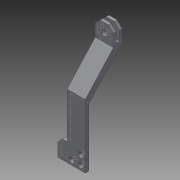
# Autodesk Inventor part: col support base
Saved by Autodesk Inventor 2015 (Build 190159000, 159)
## iProperties
Created: 2019-01-13
Part Number: col support base
Material: Generic
Document SubType Name: Modeling
Designer: Toby
Density: 1 g/cm^3
Appearance: Default
Author: Toby
Autodesk Inventor part; units mm, degrees
ref_plane "YZ Plane" through (0, 0, 0) normal (1, 0, 0) x (0, 1, 0)
ref_plane "XZ Plane" through (0, 0, 0) normal (0, 1, 0) x (-1, 0, 0)
ref_plane "XY Plane" through (0, 0, 0) normal (0, 0, 1) x (1, 0, 0)
sketch "Sketch1" plane through (0, 0, 0) normal (0, 0, 1) x (1, 0, 0)
  line L0 (-18.6815, -3.2252) -> (11.3185, -3.2252)
  line L1 (11.3185, -3.2252) -> (11.3185, -7.2252)
  line L2 (11.3185, -7.2252) -> (-18.6815, -7.2252)
  line L3 (-18.6815, -7.2252) -> (-18.6815, -3.2252)
  point P0 (0, 0)
  dimension "d0" = 30
  dimension "d1" = 4
  constraints: 8 end point, 2 parallel, 1 horizontal, 1 perpendicular
  measures "d0" distance of L0.start L0.end
  measures "d1" distance of L2.end L0.start
extrude "Extrusion1" add sketch "Sketch1" along normal blind 20
sketch "Sketch2" plane through (-18.6815, -7.2252, 0) normal (0, -1, 0) x (1, 0, 0)
  line L0 (30, 20) -> (10, 20)
  line L1 (10, 20) -> (10, 123)
  line L2 (10, 123) -> (30, 123)
  line L3 (30, 123) -> (30, 20)
  point P0 (18.6815, 0)
  dimension "d4" = 103
  dimension "d5" = 20
  constraints: 8 end point, 2 parallel, 1 horizontal, 1 perpendicular
  measures "d4" distance of L0.end L1.end
  measures "d5" distance of L1.end L2.end
extrude "Extrusion2" add sketch "Sketch2" against normal blind 10
sketch "Sketch3" plane through (-18.6815, -7.2252, 0) normal (0, -1, 0) x (1, 0, 0)
  line L0 (30, 20) -> (10, 20) projected
  line L1 (30, 0) -> (30, 20) projected
  line L2 (30, 0) -> (0, 0) projected
  point P0 (18.6815, 0)
  point P1 (25, 15)
  point P2 (25, 5)
  point P3 (15, 5)
  dimension "d8" = 5
  dimension "d9" = 5
  dimension "d10" = 5
  dimension "d11" = 5
  dimension "d12" = 5
  dimension "d13" = 10
  measures "d8" distance from line of L0 point (25, 15)
  measures "d9" distance from line of L1 point (25, 15)
  measures "d10" distance from line of L2 point (25, 5)
  measures "d11" distance from line of L1 point (25, 5)
  measures "d12" distance from line of L2 point (15, 5)
  measures "d13" distance of point (25, 5) point (15, 5)
hole "Hole1" at (6.3185, -7.2252, 15) at (6.3185, -7.2252, 5) at (-3.6815, -7.2252, 5) direction (0, 1, 0) diameter 3 depth 8 tip angle 118 countersink diameter 6 countersink angle 90
chamfer "Chamfer1" distance 5 angle 45 1 edges at (-18.6815, -5.2252, 20)
sketch "Sketch4" plane through (-8.6815, -7.2252, 20) normal (-1, 0, 0) x (0, 0, 1)
  line L0 (103, 10) -> (0, 10)
  line L1 (0, 10) -> (0, 4)
  line L2 (0, 4) -> (103, 4)
  line L3 (103, 4) -> (103, 10)
  point P0 (-20, 7.2252)
  constraints: 8 end point, 2 parallel, 1 horizontal, 1 perpendicular
extrude "Extrusion3" cut sketch "Sketch4" against normal blind 20
sketch "Sketch5" plane through (-8.6815, -7.2252, 20) normal (-1, 0, 0) x (0, 0, 1)
  line L0 (103, 4) -> (99, 4)
  line L1 (99, 4) -> (99, 34)
  line L2 (99, 34) -> (103, 34)
  line L3 (103, 34) -> (103, 4)
  point P0 (-20, 7.2252)
  dimension "d26" = 4
  dimension "d27" = 30
  constraints: 8 end point, 2 parallel, 1 horizontal, 1 perpendicular
  measures "d26" distance between parallel lines of L1 L3
  measures "d27" distance between parallel lines of L0 L2
extrude "Extrusion4" add sketch "Sketch5" against normal blind 20
sketch "Sketch6" plane through (-8.6815, -7.2252, 20) normal (-1, 0, 0) x (0, 0, 1)
  line L0 (103, 34) -> (88, 34)
  line L1 (88, 34) -> (88, 31)
  line L2 (88, 31) -> (103, 31)
  line L3 (103, 31) -> (103, 34)
  line L4 (103, 37.5) -> (88, 37.5)
  line L5 (88, 37.5) -> (88, 40.5)
  line L6 (88, 40.5) -> (103, 40.5)
  line L7 (103, 40.5) -> (103, 37.5)
  line L8 (103, 0) -> (103, 34) projected
  line L9 (88, 40.5) -> (84, 40.5)
  line L10 (84, 40.5) -> (84, 31)
  line L11 (84, 31) -> (88, 31)
  line L12 (88, 31) -> (88, 40.5)
  point P0 (-20, 7.2252)
  dimension "d30" = 15
  dimension "d31" = 3
  dimension "d32" = 3.5
  dimension "d33" = 3
  dimension "d34" = 4
  constraints: 24 end point, 6 parallel, 3 collinear, 3 horizontal, 3 perpendicular
  measures "d30" distance between parallel lines of L1 L3
  measures "d31" distance between parallel lines of L0 L2
  measures "d32" distance between parallel lines of L0 L4
  measures "d33" distance between parallel lines of L4 L6
  measures "d34" distance between parallel lines of L10 L12
extrude "Extrusion5" add sketch "Sketch6" against normal blind 20
sketch "Sketch7" plane through (-8.6815, -7.2252, 20) normal (-1, 0, 0) x (0, 0, 1)
  line L0 (88, 37.5) -> (87, 37.5)
  line L1 (87, 37.5) -> (87, 34)
  line L2 (87, 34) -> (88, 34)
  line L3 (88, 34) -> (88, 37.5)
  line L4 (103, 34) -> (88, 34) projected
  point P0 (-20, 7.2252)
  dimension "d37" = 1
  constraints: 8 end point, 2 parallel, 1 collinear, 1 horizontal, 1 perpendicular
  measures "d37" distance between parallel lines of L1 L3
extrude "Extrusion6" cut sketch "Sketch7" against normal blind 20
sketch "Sketch8" plane through (-8.6815, -7.2252, 20) normal (-1, 0, 0) x (0, 0, 1)
  line L0 (103, 34) -> (103, 0) projected
  line L1 (-20, 0) -> (103, 0) projected
  line L2 (103, 31) -> (50, 31)
  line L3 (50, 31) -> (50, 0)
  line L4 (50, 0) -> (103, 0)
  line L5 (103, 0) -> (103, 31)
  line L6 (84, 31) -> (99, 31) projected
  line L7 (0, 0) -> (0, 4) projected
  point P0 (-20, 7.2252)
  dimension "d40" = 50
  constraints: 8 end point, 2 parallel, 2 point on line, 1 collinear, 1 horizontal, 1 perpendicular
  measures "d40" distance between parallel lines of L7 L3
extrude "Extrusion7" cut sketch "Sketch8" against normal blind 20
sketch "Sketch9" plane through (11.3185, -7.2252, 0) normal (1, 0, 0) x (0, 0, -1)
  line L0 (-104, 40.5) -> (-104, 31)
  line L1 (-104, 31) -> (-104, 40.5) projected
  line L2 (-104, 31) -> (-70, 0)
  line L3 (-104, 40.5) -> (-70, 9.5)
  line L4 (-70, 9.5) -> (-70, 0)
  line L5 (-70, 4) -> (-70, 0) projected
  line L6 (-70, 9.5) -> (-59.5806, 0)
  line L7 (-59.5806, 0) -> (-70, 0)
  line L8 (0, 0) -> (-70, 0) projected
  point P0 (0, 7.2252)
  constraints: 12 end point, 3 collinear, 2 parallel
extrude "Extrusion8" add sketch "Sketch9" against normal blind 20
sketch "Sketch10" plane through (-8.6815, 23.7748, 123) normal (0, -1, 0) x (1, 0, 0)
  line L0 (0, -16) -> (20, -16) projected
  point P0 (8.6815, -123)
  point P1 (10, -10)
  dimension "d45" = 6
  measures "d45" distance from line of L0 point (10, -10)
hole "Hole2" at (1.3185, 23.7748, 113) direction (0, 1, 0) diameter 3 depth 15 tip angle 118 countersink diameter 6 countersink angle 90
chamfer "Chamfer2" distance 5.5 angle 45 4 edges at (11.3185, 31.7748, 123) (-8.6815, 31.7748, 123) (11.3185, 25.2748, 123) (-8.6815, 25.2748, 123)
body "Solid1"
